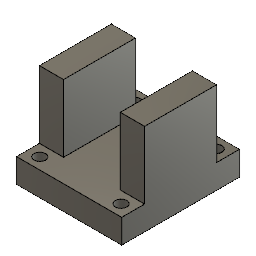
IMU Mount (Autodesk Fusion 360 design; units mm, degrees)
Autodesk Fusion 360 part; units mm, degrees
note: some values were not read from the file. Set by a fixed rule: which sketch regions a step uses.
sketch "Sketch1" plane through (0, 0, 0) normal (0, 1, 0) x (1, 0, 0)
  line L0 (0, 0) -> (12.4, 0)
  line L1 (12.4, 0) -> (12.4, -25.75)
  line L2 (12.4, -25.75) -> (0, -25.75)
  line L3 (0, -25.75) -> (0, 0)
  line L4 (0, 0) -> (-5.3, 0)
  line L5 (-5.3, 0) -> (-5.3, -25.75)
  line L6 (-5.3, -25.75) -> (0, -25.75)
  line L7 (0, -25.75) -> (0, 0)
  line L8 (12.4, 0) -> (17.7, 0)
  line L9 (17.7, 0) -> (17.7, -25.75)
  line L10 (17.7, -25.75) -> (12.4, -25.75)
  line L11 (12.4, -25.75) -> (12.4, 0)
  line L12 (-5.3, -25.75) -> (-2.675, -25.75)
  line L13 (-2.675, -25.75) -> (-2.675, -23.25)
  line L14 (-2.675, -23.25) -> (-5.3, -23.25)
  line L15 (-5.3, -23.25) -> (-5.3, -25.75)
  line L16 (-2.675, -23.25) -> (15.075, -23.25)
  line L17 (-2.675, -23.25) -> (-2.675, -2.5)
  circle A0 centre (-2.675, -23.25) radius 1.25
  circle A1 centre (-2.675, -2.5) radius 1.25
  circle A2 centre (15.075, -23.25) radius 1.25
  line L18 (-2.675, -2.5) -> (15.075, -2.5)
  circle A3 centre (15.075, -2.5) radius 1.25
  dimension "d1" = 12.4
  dimension "d2" = 25.75
  dimension "d3" = 5.3
  dimension "d4" = 5.3
  dimension "d5" = 25.75
  dimension "d6" = 25.75
  dimension "d13" = 2.625
  dimension "d14" = 2.5
  dimension "d15" = 17.75
  dimension "d16" = 20.75
  dimension "d17" = 2.5
  dimension "d18" = 2.5
  dimension "d19" = 2.5
  dimension "d20" = 17.75
  dimension "d21" = 2.5
  constraint horizontal L0
  constraint vertical L1
  constraint horizontal L2
  constraint vertical L3
  constraint coincident L0.start L3.end
  constraint horizontal L4
  constraint vertical L5
  constraint horizontal L6
  constraint vertical L7
  constraint horizontal L8
  constraint vertical L9
  constraint horizontal L10
  constraint vertical L11
  constraint horizontal L12
  constraint vertical L13
  constraint horizontal L14
  constraint vertical L15
  constraint perpendicular L13 L16
  constraint perpendicular L14 L17
  constraint coincident L13.end L14.start
  constraint coincident L17.end A1.centre
  constraint coincident L16.end A2.centre
  constraint perpendicular L11 L18
  constraint coincident L18.end A3.centre
  measures "d1" distance of L0.start L0.end
  measures "d2" distance of L0.start L2.end
  measures "d3" distance of L0.start L4.end
  measures "d4" distance of L0.end L8.end
  measures "d5" distance of L0.end L1.end
  measures "d6" distance of L4.end L5.end
  measures "d13" distance of L5.end L12.end
  measures "d14" distance of L5.end L14.end
  measures "d15" distance of L13.end L16.end
  measures "d16" distance of L13.end L17.end
  measures "d17" diameter of A0
  measures "d18" diameter of A1
  measures "d19" diameter of A2
  measures "d20" distance of L17.end L18.end
  measures "d21" diameter of A3
extrude "Extrude1" add sketch "Sketch1" along normal blind 5.3 contours L0 L1 L3 L7 L11 L18 | L3 L4 L5 L7 L14 L17 A0 A1 L18 | L1 L8 L9 L10 L11 | L1 L3 L7 L11 L16 L18 | L3 L7 L16 L17 A0 A1 L18 | L1 L2 L3 L7 L11 L16 | L3 L6 L7 L13 L16 A0 | L17 A1 L18 | L17 A1 L18 | L5 L6 L12 L13 L14 L15 A0 | L13 L16 A0 | L16 L17 A0 | L14 L17 A0 | L13 L14 A0 | A2 | A3
extrude "Extrude2" add sketch "Sketch1" along normal blind 20 contours L3 L4 L5 L7 L14 L17 A0 A1 L18 | L1 L8 L9 L10 L11 | L3 L7 L16 L17 A0 A1 L18 | L3 L6 L7 L13 L16 A0 | L17 A1 L18 | L17 A1 L18 | L5 L6 L12 L13 L14 L15 A0 | L13 L16 A0 | L16 L17 A0 | L14 L17 A0 | L13 L14 A0 | A2 | A3
extrude "Extrude3" cut sketch "Sketch1" along normal up to surface (20 mm away) contours L17 A1 L18 | L17 A1 L18 | L13 L16 A0 | L16 L17 A0 | L14 L17 A0 | L13 L14 A0 | A2 | A3
sketch "Sketch3" plane through (0, 20, 0) normal (0, 1, 0) x (-1, 0, 0)
  circle A0 centre (2.675, 23.25) radius 1.25
  circle A1 centre (2.675, 2.5) radius 1.25
  line L0 (0, 25.75) -> (0, 0)
  line L1 (0, 0) -> (5.3, 0)
  line L2 (5.3, 0) -> (5.3, 25.75)
  line L3 (5.3, 25.75) -> (0, 25.75)
  line L4 (2.675, 2.5) -> (2.675, 5)
  line L5 (2.675, 5) -> (0, 5)
  line L6 (2.675, 5) -> (5.3, 5)
  line L7 (2.675, 23.25) -> (2.675, 20.75)
  line L8 (2.675, 20.75) -> (-2, 20.75)
  line L9 (-2, 20.75) -> (2.675, 20.75)
  line L10 (7.8916, 20.75) -> (2.675, 20.75)
  dimension "d24" = 2.5
  dimension "d25" = 2.5
  constraint coincident A1.centre L4.start
  constraint perpendicular L1 L4
  constraint coincident L0 L5.end
  constraint perpendicular L0 L5
  constraint coincident L2 L6.end
  constraint perpendicular L2 L6
  constraint coincident A0.centre L7.start
  constraint perpendicular L6 L7
  constraint perpendicular L0 L8
  constraint perpendicular L7 L10
  measures "d24" distance of A1.centre L4.end
  measures "d25" distance of A0.centre L7.end
extrude "Extrude4" cut sketch "Sketch3" against normal blind 14.7 contours L0 L1 L2 L5 L6 | L0 L2 L3 L8 L9 L10
sketch "Sketch4" plane through (0, 20, 0) normal (0, 1, 0) x (-1, 0, 0)
  circle A0 centre (-15.075, 23.25) radius 1.25
  circle A1 centre (-15.075, 2.5) radius 1.25
  line L0 (-12.4, 25.75) -> (-17.7, 25.75)
  line L1 (-17.7, 25.75) -> (-17.7, 0)
  line L2 (-17.7, 0) -> (-12.4, 0)
  line L3 (-12.4, 0) -> (-12.4, 25.75)
  line L4 (-15.075, 2.5) -> (-15.075, 5)
  line L5 (-9.6971, 5) -> (-24, 5)
  line L6 (-15.075, 23.25) -> (-15.075, 20.75)
  line L7 (-20.719, 20.75) -> (-5, 20.75)
  dimension "d28" = 2.5
  dimension "d29" = 2.5
  constraint coincident A1.centre L4.start
  constraint parallel L1 L4
  constraint perpendicular L3 L5
  constraint coincident A0.centre L6.start
  constraint vertical L6
  constraint perpendicular L1 L7
  measures "d28" distance of A1.centre L4.end
  measures "d29" distance of A0.centre L6.end
extrude "Extrude5" cut sketch "Sketch4" against normal blind 14.7 contours L0 L1 L3 L7 | L1 L2 L3 L5
